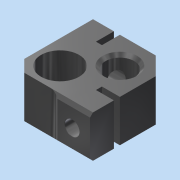
# Autodesk Inventor part: FOX-ME-118-03
Saved by Autodesk Inventor 2014 (Build 180170000, 170)
## iProperties
Created: 2011-09-05
Part Number: FOX-ME-118-03
Document SubType Name: Modeling
Designer: Robert Davis
Density: 1.41 g/cm^3
Material: Delrin, Black
Mass: 1.20114 g
Surface Area: 10.4619 cm^2
Volume: 0.85187 cm^3
Description: PCB DELRIN MOUNT
Appearance: Smooth - Medium Gray
Author: Robert Davis
Autodesk Inventor part; units mm, degrees
ref_plane "YZ Plane" through (0, 0, 0) normal (1, 0, 0) x (0, 1, 0)
ref_plane "XZ Plane" through (0, 0, 0) normal (0, 1, 0) x (-1, 0, 0)
ref_plane "XY Plane" through (0, 0, 0) normal (0, 0, 1) x (1, 0, 0)
sketch "Sketch1" plane through (0, 0, 0) normal (0, 0, 1) x (1, 0, 0)
  line L0 (0, 0) -> (14, 0)
  line L1 (14, 0) -> (14, 14)
  line L2 (14, 14) -> (0, 14)
  line L3 (0, 14) -> (0, 0)
  dimension "d0" = 14
  dimension "d1" = 14
  constraints: 8 end point, 2 horizontal, 2 vertical, 1 coincident
  measures "d0" distance of L1.end L2.end
  measures "d1" distance of L0.end L1.end
extrude "Extrusion1" add sketch "Sketch1" along normal mid plane 7
hole "Hole1" at (9.5, 9.5, 3.5) direction (0, 0, -1) diameter 4.7752 end through all
sketch "Sketch22" plane through (0, 0, 3.5) normal (0, 0, 1) x (1, 0, 0)
  line L0 (0, 0) -> (0, 14) projected
  line L1 (14, 0) -> (0, 0) projected
  arc A0 (0.5, 0) -> (0, 0.5) centre (0, 0) ccw
  line L2 (0, 0.5) -> (0, 0)
  line L3 (0, 0) -> (0.5, 0)
  dimension "d145" = 0.5
  constraints: 4 end point, 2 collinear, 2 point on circle, 1 centre point, 1 coincident
  measures "d145" radius of A0
extrude "Extrusion19" cut sketch "Sketch22" against normal through all
sketch "Sketch15" plane through (0, 0, 3.5) normal (0, 0, 1) x (1, 0, 0)
  line L0 (14, 0) -> (0, 0) projected
  line L1 (0, 0) -> (0, 14) projected
  line L2 (5, 5) -> (5, 12)
  line L3 (5, 12) -> (4, 12)
  line L4 (4, 12) -> (4, 5)
  line L5 (5, 4) -> (12, 4)
  line L6 (12, 4) -> (12, 5)
  line L7 (12, 5) -> (5, 5)
  arc A0 (0.5, 0) -> (0, 0.5) centre (0, 0) ccw projected
  line L8 (4, 5) -> (0, 5)
  line L9 (0, 5) -> (0, 0)
  line L10 (0, 0) -> (5, 0)
  line L11 (5, 0) -> (5, 4)
  point P0 (0, 7.5)
  point P1 (7.5, 0)
  point P2 (0.315, 0.3883)
  dimension "d94" = 1
  dimension "d95" = 4
  dimension "d96" = 4
  dimension "d97" = 12
  constraints: 20 end point, 5 parallel, 2 perpendicular, 1 point on circle
  measures "d94" distance of L5.end L6.end
  measures "d95" distance between parallel lines of L0 L5
  measures "d96" distance between parallel lines of L1 L4
  measures "d97" distance between parallel lines of L0 L3
extrude "sawblade" [suppressed]
chamfer "Chamfer5" distance 3 angle 45 1 edges at (14, 14, 0)
chamfer "Chamfer8" distance 0.5 angle 45 4 edges at (7.25, 0, 3.5) (0, 7.25, 3.5) (7.25, 0, -3.5) (0, 7.25, -3.5)
chamfer "Chamfer9" distance 0.5 angle 45 2 edges at (9.5, 11.8876, 3.5) (9.5, 11.8876, -3.5)
hole "Hole6" at (11, 0, 0) direction (0, 1, 0) diameter 2.4384 depth 8 tip angle 118 countersink diameter 2.54 countersink angle 120
hole "Hole7" at (0, 11, 0) direction (1, 0, 0) diameter 2.4384 depth 8 tip angle 118 countersink diameter 2.54 countersink angle 120
sketch "Sketch25" plane through (0, 0, 3.5) normal (0, 0, 1) x (1, 0, 0)
  line L0 (0.5, 14) -> (11, 14) projected
  line L1 (5, 14) -> (4, 14)
  line L2 (4, 14) -> (4, 11)
  line L3 (4, 11) -> (5, 11)
  line L4 (5, 11) -> (5, 14)
  line L5 (0, 14) -> (0, 0.5) projected
  point P0 (0, 0)
  dimension "d183" = 3
  dimension "d184" = 4
  dimension "d185" = 1
  constraints: 8 end point, 1 collinear
  measures "d183" distance of L1.end L2.end
  measures "d184" distance between parallel lines of L5 L2
  measures "d185" distance of L1.start L1.end
extrude "sawblade1" cut sketch "Sketch25" against normal through all
sketch "Sketch26" plane through (0, 0, 3.5) normal (0, 0, 1) x (1, 0, 0)
  line L0 (14, 5) -> (11, 5)
  line L1 (11, 5) -> (11, 4)
  line L2 (11, 4) -> (14, 4)
  line L3 (14, 4) -> (14, 5)
  line L4 (0.5, 0) -> (14, 0) projected
  point P0 (0, 0)
  dimension "d188" = 4
  dimension "d189" = 1
  dimension "d190" = 3
  constraints: 8 end point
  measures "d188" distance between parallel lines of L4 L2
  measures "d189" distance of L2.end L0.start
  measures "d190" distance of L1.end L2.end
extrude "sawblade2" cut sketch "Sketch26" against normal through all
hole "Hole8" [suppressed]
hole "Hole9" [suppressed]
hole "Hole10" at (4.5, 4.5, 3.5) direction (0, 0, -1) diameter 6.35 depth 5.5
sketch "Sketch27" plane through (0, 0, 3.5) normal (0, 0, 1) x (1, 0, 0)
  line L0 (2.5, 0.5) -> (6.825, 0.5)
  line L1 (10, -2.675) -> (10, -7.675)
  line L2 (10, -7.675) -> (-7.675, -7.675)
  line L3 (-7.675, -7.675) -> (-7.675, 10)
  line L4 (-7.675, 10) -> (-2.675, 10)
  arc A0 (10, -2.675) -> (6.825, 0.5) centre (6.825, -2.675) ccw
  arc A1 (0.5, 6.825) -> (-2.675, 10) centre (-2.675, 6.825) ccw
  line L5 (0.5, 2.5) -> (0.5, 6.825)
  line L6 (2.5, 0.5) -> (0.5, 2.5)
  point P0 (0, 0)
  point P1 (0.5, 0.5)
  dimension "d220" = 3.175
  dimension "d222" = 0.5
  dimension "d223" = 0.5
  dimension "d225" = 5
  dimension "d226" = 2
  dimension "d227" = 2
  dimension "d228" = 10
  constraints: 14 end point, 4 point on circle, 4 tangent, 3 horizontal, 3 vertical, 2 centre point, 2 perpendicular, 2 point on line, 1 equal radius
  measures "d220" radius of A0
  measures "d222" distance from line of point (0, 0) L5
  measures "d223" distance from line of point (0, 0) L0
  measures "d225" distance of L3.end L4.end
  measures "d226" distance of L0.start point (0.5, 0.5)
  measures "d227" distance of L5.start point (0.5, 0.5)
  measures "d228" distance from line of L1 point (0, 0)
extrude "Extrusion24" cut sketch "Sketch27" against normal through all
hole "Hole11" at (4.5, 4.5, -2) direction (0, 0, -1) diameter 3.175 end through all
equation "\"d227\" = d226"
body "Solid1"
